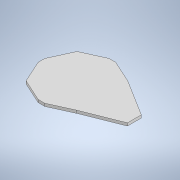
# Autodesk Inventor part: Деталь7
Saved by Autodesk Inventor 2022 (Build 260153000, 153)
## iProperties
Created: 2022-03-25
Part Number: Деталь7
Material: Типовые
Document SubType Name: Modeling
Designer: Josh
Density: 1 g/cm^3
Appearance: По умолчанию
Author: Josh
Autodesk Inventor part; units mm, degrees
ref_plane "YZ Plane" through (0, 0, 0) normal (1, 0, 0) x (0, 1, 0)
ref_plane "XZ Plane" through (0, 0, 0) normal (0, 1, 0) x (-1, 0, 0)
ref_plane "XY Plane" through (0, 0, 0) normal (0, 0, 1) x (1, 0, 0)
sketch "Эскиз1" plane through (0, 0, 0) normal (0, 1, 0) x (-1, 0, 0)
  line L0 (-44, 88) -> (-44, 96)
  line L1 (-36, 96) -> (-44, 96)
  line L2 (-44, 72) -> (-44, 80)
  line L3 (-44, 72) -> (-36, 72)
  line L4 (-7.5, 172) -> (-7.5, 176)
  line L5 (0, 176) -> (-7.5, 176)
  line L6 (72, 212) -> (72, 204)
  line L7 (72, 212) -> (80, 212)
  line L8 (88, 212) -> (96, 212)
  line L9 (96, 204) -> (96, 212)
  line L10 (172, 175.5) -> (176, 175.5)
  line L11 (176, 168) -> (176, 175.5)
  line L12 (212, 96) -> (204, 96)
  line L13 (212, 96) -> (212, 88)
  line L14 (212, 80) -> (212, 72)
  line L15 (204, 72) -> (212, 72)
  line L16 (175.5, -4) -> (175.5, -8)
  line L17 (168, -8) -> (175.5, -8)
  line L18 (96, -44) -> (88, -44)
  line L19 (96, -44) -> (96, -36)
  line L20 (80, -44) -> (72, -44)
  line L21 (72, -36) -> (72, -44)
  line L22 (-4, -7.5) -> (-8, -7.5)
  line L23 (-8, 0) -> (-8, -7.5)
  line L24 (-44, 72) -> (-8, -7.5)
  line L25 (-8, -7.5) -> (72, -44)
  line L26 (96, -44) -> (175.5, -8)
  line L27 (212, 72) -> (175.5, -8)
  line L28 (212, 96) -> (176, 175.5)
  line L29 (176, 175.5) -> (96, 212)
  line L30 (72, 212) -> (-7.5, 176)
  line L31 (-7.5, 176) -> (-44, 96)
  line L32 (72, 212) -> (96, 212)
  line L33 (212, 96) -> (212, 72)
  line L34 (96, -44) -> (72, -44)
  line L35 (-44, 72) -> (-44, 96)
  line L36 (-133.5, 90) -> (-133.5, 78)
  line L37 (-8, -7.5) -> (-138.5, 74)
  line L38 (-138.5, 74) -> (-138.5, 124)
  line L39 (-138.5, 124) -> (-7.5, 176)
  point P0 (0, 0)
  constraints: 80 end point, 8 perpendicular, 2 vertical, 1 horizontal
extrude "Выдавливание1" add sketch "Эскиз1" along normal blind 10
